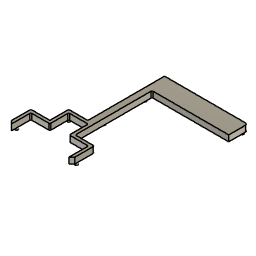
ROYAL_KLUDGE_96_Volume_Cover (Autodesk Fusion 360 design; units mm, degrees)
Autodesk Fusion 360 part; units mm, degrees
sketch "Sketch2" plane through (0, 0, 0) normal (0, 0, 1) x (1, 0, 0)
  line L0 (0, 19.2) -> (0, 0)
  line L1 (83.4995, 0.3) -> (6.3, 0.3)
  line L2 (0, -58) -> (0, 19.2)
  line L3 (83.4995, 0.3) -> (84.0001, 0.3)
  line L4 (25.45, -77) -> (6.3, -77)
  line L5 (6.3, -77) -> (6.3, 0.3)
  circle A0 centre (3.15, -44.9767) radius 1.5
  circle A1 centre (3.15, -3.7) radius 1.5
  circle A2 centre (80.7, 16.6) radius 1.5
  circle A3 centre (-36.85, -92.9) radius 1.5
  line L6 (25.45, -77) -> (25.45, -96.5)
  line L7 (-16.2, -61) -> (3.3, -61)
  line L8 (3.3, -61) -> (3.3, -80)
  line L9 (3.3, -80) -> (22.45, -80)
  line L10 (22.45, -80) -> (22.45, -99.5)
  line L11 (22.45, -99.5) -> (25.45, -96.5)
  circle A4 centre (23.95, -93.4) radius 1.5
  circle A5 centre (-17.3909, -59.7422) radius 1.5
  line L12 (3.1245, 19.3) -> (3.1245, -34.9) construction
  line L13 (23.85, -77) -> (23.85, -78.6) construction
  line L14 (-37.25, -77) -> (-37.25, -78.6) construction
  line L15 (0, -58) -> (-19.2, -58)
  line L16 (-19.2, -58) -> (-19.2, -77)
  line L17 (-19.2, -77) -> (-38.35, -77)
  line L18 (-38.35, -77) -> (-38.35, -96.5)
  line L19 (-16.2, -61) -> (-16.2, -80)
  line L20 (-16.2, -80) -> (-35.35, -80)
  line L21 (-35.35, -80) -> (-35.35, -99.5)
  line L22 (-38.35, -96.5) -> (-35.35, -99.5)
  line L23 (83.4995, 0.3) -> (83.4995, 19.2)
  line L24 (0, 19.2) -> (83.4995, 19.2)
  dimension "d1" = 83.5
  dimension "d2" = 19.2
  dimension "d28" = 3
  dimension "d30" = 23
  dimension "d31" = 3
  dimension "d35" = 3
  dimension "d38" = 3
  dimension "d44" = 19.5
  dimension "d46" = 19.5
  dimension "d47" = 19
  dimension "d48" = 19.15
  dimension "d49" = 19.5
  dimension "d51" = 3
  dimension "d52" = 3
  dimension "d61" = 54.2
  dimension "d63" = 1.6
  dimension "d65" = 1.6
  dimension "d90" = 19.2
  dimension "d91" = 19.15
  dimension "d92" = 19.5
  dimension "d93" = 19.15
  dimension "d94" = 19.5
  dimension "d101" = 18.9
  constraint vertical L0
  constraint coincident L0.end origin
  constraint coincident L1 L3.end
  constraint perpendicular L1 L5
  constraint perpendicular L4 L6
  constraint perpendicular L7 L8
  constraint perpendicular L8 L9
  constraint perpendicular L9 L10
  constraint vertical L12
  constraint perpendicular L4 L13
  constraint perpendicular L17 L18
  constraint perpendicular L19 L20
  constraint perpendicular L20 L21
  constraint perpendicular L3 L23
  constraint perpendicular L23 L24
  measures "d1" distance of L0.end L1.start
  measures "d2" distance of L0.end L0.start
  measures "d28" diameter of A0
  measures "d30" distance of L12.start A1.centre
  measures "d31" diameter of A1
  measures "d35" diameter of A2
  measures "d38" diameter of A3
  measures "d44" distance of L4.start L6.end
  measures "d46" distance of L7.start L7.end
  measures "d47" distance of L7.end L8.end
  measures "d48" distance of L8.end L9.end
  measures "d49" distance of L9.end L10.end
  measures "d51" diameter of A4
  measures "d52" diameter of A5
  measures "d61" distance of L12.start L12.end
  measures "d63" distance of L13.start L13.end
  measures "d65" distance of L14.start L14.end
  measures "d90" distance of L2.start L15.end
  measures "d91" distance of L16.end L17.end
  measures "d92" distance of L17.end L18.end
  measures "d93" distance of L19.end L20.end
  measures "d94" distance of L20.end L21.end
  measures "d101" distance of L1.start L23.end
extrude "Extrude1" add sketch "Sketch2" along normal blind 6 contours L0 L1 L2 L4 L5 A3 L6 L7 L8 L9 L10 A4 L15 L16 L17 L18 L19 L20 L21 L23 L24 | A3 | A3 L18 L21 L22 | A4 | L6 L10 L11 A4 | A0 | A1 | A2 | A5
extrude "Extrude2" add sketch "Sketch2" against normal blind 2.4 contours A3 | A4 | A0 | A1 | A2 | A5
fillet "Fillet1" radius 1 12 edges at (3.3, -80, 3) (25.45, -77, 3) (22.45, -80, 3) (3.3, -61, 3) (6.3, 0.3, 3) (-38.35, -77, 3) (-16.2, -80, 3) (-35.35, -80, 3) (-16.2, -61, 3) (-19.2, -58, 3) (0, -58, 3) (6.3, -77, 3)
fillet "Fillet1" radius 2 1 edges at (83.4995, 19.2, 3)
equation "d53 = height"
equation "screw_hole_diameter = 1.8 mm"
equation "screw_hole_depth = height - 1.5 mm"
equation "height = 6 mm"
